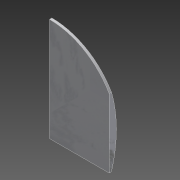
# Autodesk Inventor part: palmrest
Saved by Autodesk Inventor 2018 (Build 220112000, 112)
## iProperties
Created: 2018-07-06
Part Number: palmrest
Material: ABS プラスチック
Document SubType Name: モデリング
Designer: NaMACHAN
Mass: 29.2311 g
Surface Area: 123.438 cm^2
Volume: 10.8263 cm^3
Density: 1.06 g/cm^3
Appearance: 滑らか - 白
Sheet Metal Width: 0.000 mm
Sheet Metal Length: 0.000 mm
Sheet Metal Area: 0.000 mm^2
Author: NaMACHAN
Autodesk Inventor part; units mm, degrees
ref_plane "YZ Plane" through (0, 0, 0) normal (1, 0, 0) x (0, 1, 0)
ref_plane "XZ Plane" through (0, 0, 0) normal (0, 1, 0) x (-1, 0, 0)
ref_plane "XY Plane" through (0, 0, 0) normal (0, 0, 1) x (1, 0, 0)
sketch "スケッチ19" plane through (0, 0, 0) normal (1, 0, 0) x (0, 1, 0)
  arc A0 (0, -150) -> (150, 0) centre (0, 0) ccw
  line L0 (150, 0) -> (120, 0)
  line L1 (120, 0) -> (120, -90)
  dimension "d127" = 30
  dimension "d128" = 0
  dimension "d134" = 90
  constraints: 4 end point, 4 point on circle, 1 centre point, 1 coincident, 1 horizontal, 1 horizontal alignment, 1 perpendicular
  measures "d127" distance of L0.start L0.end
  measures "d128" distance from line of A0.end L0
  measures "d134" distance of L0.end L1.end
revolve "回転1" add sketch "スケッチ19" angle 360 about axis through (0, 150, 0) along (0, -1, 0)
sketch "スケッチ20" plane through (0, 120, 0) normal (0, -1, 0) x (0, 0, 1)
  circle A0 centre (0, 0) radius 90 projected
  line L0 (-80.6226, 40) -> (19.3774, 40)
  line L1 (19.3774, 40) -> (19.3774, -40)
  line L2 (19.3774, -40) -> (-80.6226, -40)
  line L3 (-80.6226, -40) -> (-80.6226, 40)
  dimension "d141" = 80
  dimension "d142" = 100
  constraints: 8 end point, 2 parallel, 2 point on circle, 1 horizontal, 1 perpendicular
  measures "d141" distance of L2.end L0.start
  measures "d142" distance of L1.end L2.end
extrude "押し出し5" cut sketch "スケッチ20" against normal blind 50 contours L0 L1 L2 L3 keep common part
sketch "スケッチ22" plane through (-40, 120, 19.3774) normal (0, -1, 0) x (1, 0, 0)
  line L0 (80, 0) -> (80, -100) projected
  line L1 (0, 0) -> (80, 0) projected
  line L2 (0, -100) -> (0, 0) projected
  line L3 (80, -100) -> (0, -100) projected
  point P0 (40, -19.3774)
extrude "押し出し7" add sketch "スケッチ22" along normal blind 5
fillet "フィレット2" radius 4 5 edges at (20.2616, 124.8578, -80.6226) (-20.2616, 124.8578, -80.6226) (40, 140.8082, -32.7573) (-40, 140.8082, -32.7573) (0, 148.7431, 19.3774)
sketch "スケッチ25" plane through (-40, 115, 19.3774) normal (0, -1, 0) x (1, 0, 0)
  circle A0 centre (66.8818, -99.5363) radius 3 projected
  circle A1 centre (10, -93.5578) radius 3 projected
  circle A2 centre (66.8818, -99.5363) radius 6
  circle A3 centre (10, -93.5578) radius 6
  point P0 (40, -19.3774)
  dimension "d166" = 12
  dimension "d167" = 12
  constraints: 2 centre point, 2 coincident
  measures "d166" diameter of A2
  measures "d167" diameter of A3
extrude "押し出し9" cut sketch "スケッチ25" against normal blind 10 contours A0 | A1 | A2 | A3
sketch "スケッチ26" plane through (-40, 115, 19.3774) normal (0, -1, 0) x (1, 0, 0)
  circle A0 centre (22.4419, -91.849) radius 1.5 projected
  circle A1 centre (42.3324, -93.9395) radius 1.5 projected
  circle A2 centre (71.5796, -16.5729) radius 1.5 projected
  circle A3 centre (9.9192, -10.0921) radius 1.5 projected
  point P0 (40, -19.3774)
hole "穴8" at (31.5796, 115, 2.8045) at (-30.0808, 115, 9.2853) at (2.3324, 115, -74.5621) at (-17.5581, 115, -72.4716) direction (0, 1, 0) diameter 6 end through all
sketch "スケッチ28" plane through (-40, 115, 19.3774) normal (0, -1, 0) x (1, 0, 0)
  circle A0 centre (42.3324, -93.9395) radius 3 projected
  circle A1 centre (22.4419, -91.849) radius 3 projected
  circle A2 centre (71.5796, -16.5729) radius 3 projected
  circle A3 centre (9.9192, -10.0921) radius 3 projected
  circle A4 centre (71.5796, -16.5729) radius 1.6
  circle A5 centre (9.9192, -10.0921) radius 1.6
  circle A6 centre (22.4419, -91.849) radius 1.6
  circle A7 centre (42.3324, -93.9395) radius 1.6
  circle A8 centre (42.3324, -93.9395) radius 3
  circle A9 centre (22.4419, -91.849) radius 3
  circle A10 centre (9.9192, -10.0921) radius 3
  circle A11 centre (71.5796, -16.5729) radius 3
  point P0 (40, -19.3774)
  dimension "d177" = 3.2
  dimension "d178" = 3.2
  dimension "d179" = 3.2
  dimension "d180" = 3.2
  constraints: 8 centre point, 8 coincident, 4 concentric
  measures "d177" diameter of A4
  measures "d178" diameter of A5
  measures "d179" diameter of A6
  measures "d180" diameter of A7
extrude "押し出し10" add sketch "スケッチ28" against normal blind 10
equation "\"BendRadius\" = Thickness"
equation "\"BendReliefWidth\" = Thickness"
equation "\"BendReliefDepth\" = 0.5 * Thickness"
equation "\"CornerReliefSize\" = 4 * Thickness"
equation "\"MinimumRemnant\" = 2 * Thickness"
equation "\"TransitionRadius\" = BendRadius"
equation "\"JacobiRadiusSize\" = Thickness"
equation "\"GapSize\" = Thickness"
equation "\"Thickness\" = 2"
